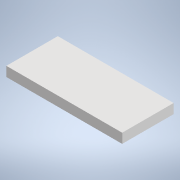
# Autodesk Inventor part: woodForkSupportBase
Saved by Autodesk Inventor 2021 (Build 250183000, 183)
## iProperties
Created: 2020-07-02
Part Number: woodForkSupportBase
Material: Generic
Document SubType Name: Modeling
Designer: robst
Density: 1 g/cm^3
Appearance: Default
Author: robst
Autodesk Inventor part; units mm, degrees
ref_plane "YZ Plane" through (0, 0, 0) normal (1, 0, 0) x (0, 1, 0)
ref_plane "XZ Plane" through (0, 0, 0) normal (0, 1, 0) x (-1, 0, 0)
ref_plane "XY Plane" through (0, 0, 0) normal (0, 0, 1) x (1, 0, 0)
sketch "Sketch1" plane through (0, 0, 0) normal (0, 1, 0) x (-1, 0, 0)
  line L0 (114.3, 50.8) -> (-114.3, 50.8)
  line L1 (-114.3, 50.8) -> (-114.3, -50.8)
  line L2 (-114.3, -50.8) -> (114.3, -50.8)
  line L3 (114.3, -50.8) -> (114.3, 50.8)
  line L4 (114.3, 50.8) -> (-114.3, -50.8) construction
  line L5 (-114.3, 50.8) -> (114.3, -50.8) construction
  point P0 (0, 0)
  dimension "d0" = 101.6
  dimension "d1" = 228.6
  constraints: 12 end point, 2 midpoint, 2 parallel, 1 horizontal, 1 perpendicular
  measures "d0" distance of L2.end L0.start
  measures "d1" distance of L0.start L0.end
extrude "Extrusion1" add sketch "Sketch1" against normal blind 19.05
body "Solid1"
